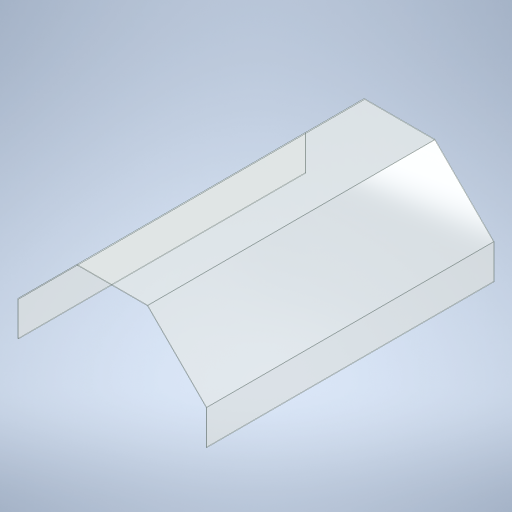
# Autodesk Inventor part: Drywall
Saved by Autodesk Inventor 2024 (Build 280153000, 153)
## iProperties
Created: 2023-05-20
Part Number: Drywall
Material: Concrete
Document SubType Name: Modeling
Designer: Tom
Density: 2.40731 g/cm^3
Appearance: Clear
Author: Tom
Autodesk Inventor part; units mm, degrees
ref_plane "YZ Plane" through (0, 0, 0) normal (1, 0, 0) x (0, 1, 0)
ref_plane "XZ Plane" through (0, 0, 0) normal (0, 1, 0) x (-1, 0, 0)
ref_plane "XY Plane" through (0, 0, 0) normal (0, 0, 1) x (1, 0, 0)
sketch "Sketch1" plane through (0, 0, 0) normal (0, 0, 1) x (1, 0, 0)
  line L0 (-2435.6949, 0) -> (-2435.6949, 895.3501)
  line L1 (-2435.6949, 895.3501) -> (-911.6949, 2419.3501)
  line L2 (-911.6949, 2419.3501) -> (911.6949, 2419.3501)
  line L3 (911.6949, 2419.3501) -> (2435.6949, 895.3501)
  line L4 (2435.6949, 895.3501) -> (2435.6949, 0)
  line L5 (903.8041, 2400.3001) -> (-903.8041, 2400.3001)
  line L6 (-903.8041, 2400.3001) -> (-2416.6449, 887.4594)
  line L7 (-2416.6449, 887.4594) -> (-2416.6449, 0)
  line L8 (2416.6449, 0) -> (2416.6449, 887.4594)
  line L9 (2416.6449, 887.4594) -> (903.8041, 2400.3001)
  line L10 (2416.6449, 0) -> (2435.6949, 0)
  line L11 (-2435.6949, 0) -> (-2416.6449, 0)
  line L12 (2435.6949, 0) -> (-2435.6949, 0)
  point P0 (0, 0)
  point P1 (0, 0)
  point P2 (0, 0)
  dimension "d2" = 4871.3898
  dimension "d3" = 135
  dimension "d4" = 1823.3898
  dimension "d5" = 19.05
  dimension "d8" = 895.3501
  dimension "d9" = 135
  dimension "d10" = 19.05
  dimension "d11" = 19.05
  dimension "d12" = 19.05
  dimension "d13" = 135
  constraints: 26 end point, 5 equal length, 2 coincident, 2 horizontal, 1 midpoint, 1 other
  measures "d2" distance of L4.end L0.start
  measures "d3" angle of L0 L1
  measures "d4" distance of L1.end L2.end
  measures "d5" distance between parallel lines of L1 L6
  measures "d8" distance of L0.start L0.end
  measures "d9" angle of L8 L9
  measures "d10" distance between parallel lines of L3 L9
  measures "d11" distance between parallel lines of L4 L8
  measures "d12" distance between parallel lines of L0 L7
  measures "d13" angle of L9 L5
extrude "Extrusion1" add sketch "Sketch1" along normal blind 7404.1 contours L0 L1 L2 L3 L4 L10 L8 L9 L5 L6 L7 L11
body "Solid1"
